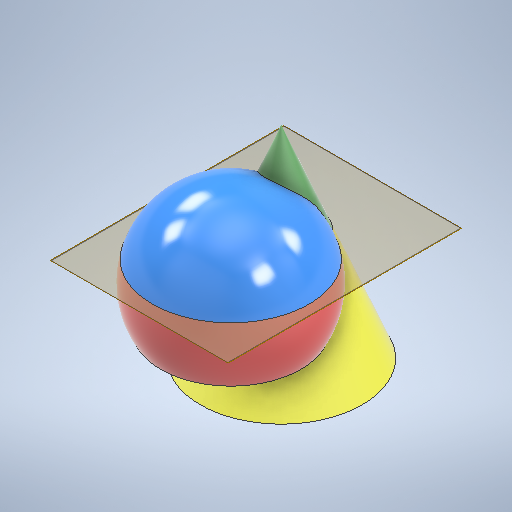
# Autodesk Inventor part: Деталь1
Saved by Autodesk Inventor 2025 (Build 290162000, 162)
## iProperties
Created: 2024-11-01
Part Number: Деталь1
Material: Типовые
Document SubType Name: Modeling
Designer: shoptick
Density: 1 g/cm^3
Appearance: По умолчанию
Mass: 340.609 g
Surface Area: 494.314 cm^2
Volume: 340.609 cm^3
Author: shoptick
Autodesk Inventor part; units mm, degrees
ref_plane "YZ Plane" through (0, 0, 0) normal (1, 0, 0) x (0, 1, 0)
ref_plane "XY Plane" through (0, 0, 0) normal (0, 0, 1) x (1, 0, 0)
sketch "Эскиз1" plane through (0, 0, 0) normal (0, 0, 1) x (1, 0, 0)
  line L0 (0, 0) -> (40, 0)
  line L1 (0, 0) -> (0, 100)
  line L2 (0, 100) -> (40, 0)
  dimension "d0" = 40
  dimension "d1" = 100
  constraints: 6 end point, 1 horizontal, 1 vertical
  measures "d0" distance of L0.start L0.end
  measures "d1" distance of L0.start L1.end
revolve "Вращение1" add sketch "Эскиз1" angle 360 about axis through (0, 0, 0) along (0, 1, 0)
sketch "Эскиз3" plane through (0, 0, 0) normal (1, 0, 0) x (0, 1, 0)
  line L0 (0, -40) -> (0, 40) projected
  arc A0 (85, 25) -> (25, 59.641) centre (45, 25) ccw
  line L1 (25, 59.641) -> (25, 25)
  line L2 (85, 25) -> (25, 25)
  point P0 (0, 0)
  dimension "d10" = 80
  constraints: 4 end point, 2 point on circle, 1 centre point, 1 horizontal
  measures "d10" diameter of A0
revolve "Вращение2" add sketch "Эскиз3" angle 360 about axis through (0, 85, 25) along (0, -1, 0)
ref_plane "РабПлоскость1" through (0, 55, 0) normal (0, 1, 0) x (-1, 0, 0)
sketch "Эскиз4" plane through (0, 55, 0) normal (0, 1, 0) x (-1, 0, 0)
  line L0 (43.5884, -45.0317) -> (-43.7808, -45.0317)
  line L1 (-43.7808, -45.0317) -> (-43.7808, 70.2418)
  line L2 (-43.7808, 70.2418) -> (43.5884, 70.2418)
  line L3 (43.5884, 70.2418) -> (43.5884, -45.0317)
  point P0 (0, 0)
  constraints: 8 end point, 2 parallel, 1 horizontal, 1 perpendicular
extrude "Выдавливание1" add sketch "Эскиз4" along normal blind 0.1 separate body
split_face "Разделение1"
split_face "Разделение2"
